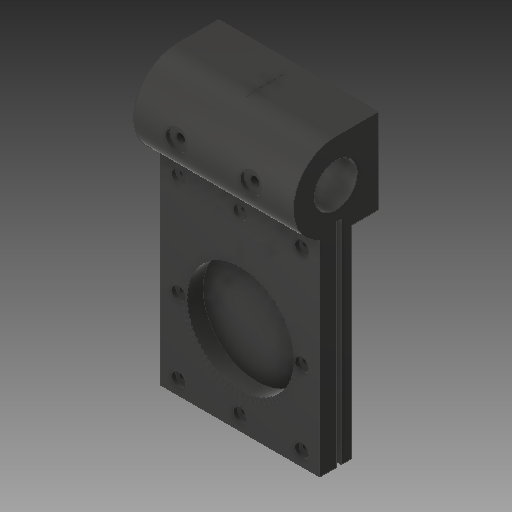
# Autodesk Inventor part: cam_holder_wrist_part
Saved by Autodesk Inventor 2019 (Build 230136000, 136)
## iProperties
Created: 2024-08-06
Part Number: cam_holder_wrist_part
Material: Acetalharz, Schwarz
Document SubType Name: Modeling
Designer: nic
Density: 1.425 g/cm^3
Appearance: Glatt - Schwarz
Author: nic
Autodesk Inventor part; units mm, degrees
(part 1 of 2)
ref_plane "YZ Plane" through (0, 0, 0) normal (1, 0, 0) x (0, 1, 0)
ref_plane "XZ Plane" through (0, 0, 0) normal (0, 1, 0) x (-1, 0, 0)
sketch "Skizze25" plane through (0, 0, 0) normal (1, 0, 0) x (0, 1, 0)
  line L0 (0, 7.5) -> (95, 7.5)
  line L1 (95, -7.5) -> (0, -7.5)
  line L2 (35.3333, -2.65) -> (95, -7.125) construction
  line L3 (100, 0) -> (115, 0) construction
  circle A0 centre (115, 0) radius 10.1
  line L4 (95, -20) -> (135, -20)
  line L5 (135, -20) -> (135, 0)
  line L6 (129.1421, 14.1421) -> (95, -20) construction
  line L7 (100.8579, 14.1421) -> (135, -20) construction
  line L8 (95, -7.125) -> (95, -20)
  line L9 (0, -2.65) -> (100, -2.65)
  line L10 (100, -2.65) -> (100, 2.65)
  line L11 (100, 2.65) -> (0, 2.65)
  line L12 (-100, 2.65) -> (-100, -2.65)
  line L13 (95, 2.5175) -> (100, 2.65) construction
  line L14 (100, -2.65) -> (95, -2.5175) construction
  line L15 (0, 7.5) -> (0, 2.65)
  line L16 (0, -2.65) -> (0, -7.5)
  arc A1 (95.1596, -2.5217) -> (95.1763, -2.65) centre (115, 0) ccw
  line L17 (95, 7.5) -> (96.4595, 7.5)
  arc A2 (135, 0) -> (96.4595, 7.5) centre (115, 0) ccw
  arc A3 (95.1763, 2.65) -> (95.1596, 2.5217) centre (115, 0) ccw
  point P0 (0, 0)
  constraints: 36 end point, 10 point on line, 8 point on circle, 4 centre point, 4 parallel, 3 horizontal, 2 coincident, 1 perpendicular, 1 tangent
extrude "Extrusion21" add sketch "Skizze25" along normal mid plane 75
sketch "Skizze26" plane through (-37.5, 0, 7.5) normal (0, 0, 1) x (1, 0, 0)
  line L0 (37.5, 96.4548) -> (37.5, 41.4548) construction
  circle A0 centre (37.5, 41.4548) radius 25.15
  point P0 (37.5, 0)
  dimension "d109" = 55
  dimension "d110" = 50.3
  constraints: 2 end point, 1 centre point, 1 coincident, 1 vertical
  measures "d109" distance of L0.start L0.end
  measures "d110" diameter of A0
extrude "Extrusion22" cut sketch "Skizze26" against normal up to surface (4.85 mm away)
ref_plane "Arbeitsebene4" through (37.5, 135, 20) normal (0, 0, -1) x (-1, 0, 0)
sketch "Skizze27" plane through (37.5, 135, 20) normal (0, 0, -1) x (-1, 0, 0)
  line L0 (75, -38.5405) -> (0, -38.5405) construction
  line L1 (0, 0) -> (0, -38.5405) construction
  line L2 (75, 0) -> (0, 0) construction
  line L3 (75, -38.5405) -> (75, 0) construction
  line L4 (75, -9.9) -> (75, -30.1) projected
  line L5 (75, -19.2702) -> (0, -19.2702)
  line L6 (75, 0) -> (0, 0) projected
  line L7 (75, 0) -> (55, 0)
  line L8 (0, 0) -> (20, 0)
  point P0 (37.5, -135)
  point P1 (55, -19.2702)
  point P2 (20, -19.2702)
  dimension "d114" = 20
  dimension "d115" = 20
  constraints: 6 end point, 5 point on line, 1 midpoint
  measures "d114" distance of L2.start L7.end
  measures "d115" distance of L1.start L8.end
hole "Bohrung2" at (-17.5, 115.7298, 20) at (17.5, 115.7298, 20) direction (0, 0, -1) diameter 4.2 depth 10 tip angle 118 counterbore diameter 10 counterbore depth 2
sketch "Skizze28" plane through (-37.5, 0, 7.5) normal (0, 0, 1) x (1, 0, 0)
  circle A0 centre (37.5, 41.4548) radius 25.15 construction
  line L0 (8.5, -6.0452) -> (66.5, -6.0452) construction
  line L1 (66.5, -6.0452) -> (66.5, 88.9548) construction
  line L2 (66.5, 88.9548) -> (8.5, 88.9548) construction
  line L3 (8.5, 88.9548) -> (8.5, -6.0452) construction
  line L4 (8.5, -6.0452) -> (66.5, 88.9548) construction
  line L5 (66.5, -6.0452) -> (8.5, 88.9548) construction
  point P0 (37.5, 0)
  point P1 (37.5, 88.9548)
  point P2 (8.5, 41.4548)
  point P3 (66.5, 41.4548)
  point P4 (8.5, 6.4399)
  point P5 (37.5, 6.4399)
  point P6 (66.5, 6.4399)
  dimension "d123" = 58
  dimension "d124" = 95
  constraints: 12 end point, 5 midpoint, 2 coincident, 2 parallel, 2 point on line, 1 horizontal, 1 perpendicular
  measures "d123" distance of L2.end L1.end
  measures "d124" distance of L1.end L0.end
hole "Bohrung3" at (0, 88.9548, 7.5) at (-29, 88.9548, 7.5) at (29, 88.9548, 7.5) at (-29, 41.4548, 7.5) at (29, 41.4548, 7.5) at (-29, 6.4399, 7.5) at (0, 6.4399, 7.5) at (29, 6.4399, 7.5) direction (0, 0, -1) diameter 3.2 end through all counterbore diameter 6.5 counterbore depth 2
sketch "Skizze29" plane through (-37.5, 0, 7.5) normal (0, 0, 1) x (1, 0, 0)
  circle A0 centre (37.5, 41.4548) radius 25.15 projected
  line L0 (37.25, 64.1048) -> (37.75, 64.1048)
  line L1 (37.75, 64.1048) -> (37.75, 69.1048)
  line L2 (37.75, 69.1048) -> (37.25, 69.1048)
  line L3 (37.25, 69.1048) -> (37.25, 64.1048)
  line L4 (37.25, 64.1048) -> (37.75, 69.1048) construction
  line L5 (37.75, 64.1048) -> (37.25, 69.1048) construction
  line L6 (35.2769, 63.9968) -> (35.775, 64.0404)
  line L7 (35.775, 64.0404) -> (35.3392, 69.0214)
  line L8 (35.3392, 69.0214) -> (34.8411, 68.9778)
  line L9 (34.8411, 68.9778) -> (35.2769, 63.9968)
  line L10 (35.2769, 63.9968) -> (35.3392, 69.0214) construction
  line L11 (35.775, 64.0404) -> (34.8411, 68.9778) construction
  line L12 (33.3207, 63.7173) -> (33.8131, 63.8041)
  line L13 (33.8131, 63.8041) -> (32.9448, 68.7282)
  line L14 (32.9448, 68.7282) -> (32.4524, 68.6413)
  line L15 (32.4524, 68.6413) -> (33.3207, 63.7173)
  line L16 (33.3207, 63.7173) -> (32.9448, 68.7282) construction
  line L17 (33.8131, 63.8041) -> (32.4524, 68.6413) construction
  line L18 (31.3963, 63.2683) -> (31.8792, 63.3977)
  line L19 (31.8792, 63.3977) -> (30.5851, 68.2274)
  line L20 (30.5851, 68.2274) -> (30.1022, 68.098)
  line L21 (30.1022, 68.098) -> (31.3963, 63.2683)
  line L22 (31.3963, 63.2683) -> (30.5851, 68.2274) construction
  line L23 (31.8792, 63.3977) -> (30.1022, 68.098) construction
  line L24 (29.5183, 62.6533) -> (29.9882, 62.8244)
  line L25 (29.9882, 62.8244) -> (28.2781, 67.5228)
  line L26 (28.2781, 67.5228) -> (27.8082, 67.3518)
  line L27 (27.8082, 67.3518) -> (29.5183, 62.6533)
  line L28 (29.5183, 62.6533) -> (28.2781, 67.5228) construction
  line L29 (29.9882, 62.8244) -> (27.8082, 67.3518) construction
  line L30 (27.7011, 61.877) -> (28.1543, 62.0883)
  line L31 (28.1543, 62.0883) -> (26.0412, 66.6199)
  line L32 (26.0412, 66.6199) -> (25.588, 66.4086)
  line L33 (25.588, 66.4086) -> (27.7011, 61.877)
  line L34 (27.7011, 61.877) -> (26.0412, 66.6199) construction
  line L35 (28.1543, 62.0883) -> (25.588, 66.4086) construction
  line L36 (25.9585, 60.9453) -> (26.3915, 61.1953)
  line L37 (26.3915, 61.1953) -> (23.8915, 65.5254)
  line L38 (23.8915, 65.5254) -> (23.4585, 65.2754)
  line L39 (23.4585, 65.2754) -> (25.9585, 60.9453)
  line L40 (25.9585, 60.9453) -> (23.8915, 65.5254) construction
  line L41 (26.3915, 61.1953) -> (23.4585, 65.2754) construction
  line L42 (24.3037, 59.8652) -> (24.7133, 60.152)
  line L43 (24.7133, 60.152) -> (21.8454, 64.2478)
  line L44 (21.8454, 64.2478) -> (21.4358, 63.961)
  line L45 (21.4358, 63.961) -> (24.3037, 59.8652)
  line L46 (24.3037, 59.8652) -> (21.8454, 64.2478) construction
  line L47 (24.7133, 60.152) -> (21.4358, 63.961) construction
  line L48 (22.7493, 58.645) -> (23.1324, 58.9664)
  line L49 (23.1324, 58.9664) -> (19.9184, 62.7966)
  line L50 (19.9184, 62.7966) -> (19.5354, 62.4752)
  line L51 (19.5354, 62.4752) -> (22.7493, 58.645)
  line L52 (22.7493, 58.645) -> (19.9184, 62.7966) construction
  line L53 (23.1324, 58.9664) -> (19.5354, 62.4752) construction
  line L54 (21.3073, 57.294) -> (21.6608, 57.6476)
  line L55 (21.6608, 57.6476) -> (18.1253, 61.1831)
  line L56 (18.1253, 61.1831) -> (17.7717, 60.8295)
  line L57 (17.7717, 60.8295) -> (21.3073, 57.294)
  line L58 (21.3073, 57.294) -> (18.1253, 61.1831) construction
  line L59 (21.6608, 57.6476) -> (17.7717, 60.8295) construction
  line L60 (19.9884, 55.8224) -> (20.3098, 56.2055)
  line L61 (20.3098, 56.2055) -> (16.4796, 59.4194)
  line L62 (16.4796, 59.4194) -> (16.1582, 59.0364)
  line L63 (16.1582, 59.0364) -> (19.9884, 55.8224)
  line L64 (19.9884, 55.8224) -> (16.4796, 59.4194) construction
  line L65 (20.3098, 56.2055) -> (16.1582, 59.0364) construction
  line L66 (18.8028, 54.2415) -> (19.0896, 54.6511)
  line L67 (19.0896, 54.6511) -> (14.9938, 57.519)
  line L68 (14.9938, 57.519) -> (14.7071, 57.1094)
  line L69 (14.7071, 57.1094) -> (18.8028, 54.2415)
  line L70 (18.8028, 54.2415) -> (14.9938, 57.519) construction
  line L71 (19.0896, 54.6511) -> (14.7071, 57.1094) construction
  line L72 (17.7595, 52.5633) -> (18.0095, 52.9963)
  line L73 (18.0095, 52.9963) -> (13.6794, 55.4963)
  line L74 (13.6794, 55.4963) -> (13.4294, 55.0633)
  line L75 (13.4294, 55.0633) -> (17.7595, 52.5633)
  line L76 (17.7595, 52.5633) -> (13.6794, 55.4963) construction
  line L77 (18.0095, 52.9963) -> (13.4294, 55.0633) construction
  line L78 (16.8665, 50.8005) -> (17.0778, 51.2537)
  line L79 (17.0778, 51.2537) -> (12.5462, 53.3668)
  line L80 (12.5462, 53.3668) -> (12.3349, 52.9136)
  line L81 (12.3349, 52.9136) -> (16.8665, 50.8005)
  line L82 (16.8665, 50.8005) -> (12.5462, 53.3668) construction
  line L83 (17.0778, 51.2537) -> (12.3349, 52.9136) construction
  line L84 (16.1305, 48.9666) -> (16.3015, 49.4365)
  line L85 (16.3015, 49.4365) -> (11.603, 51.1466)
  line L86 (11.603, 51.1466) -> (11.432, 50.6767)
  line L87 (11.432, 50.6767) -> (16.1305, 48.9666)
  line L88 (16.1305, 48.9666) -> (11.603, 51.1466) construction
  line L89 (16.3015, 49.4365) -> (11.432, 50.6767) construction
  line L90 (15.5571, 47.0756) -> (15.6865, 47.5585)
  line L91 (15.6865, 47.5585) -> (10.8569, 48.8526)
  line L92 (10.8569, 48.8526) -> (10.7274, 48.3697)
  line L93 (10.7274, 48.3697) -> (15.5571, 47.0756)
  line L94 (15.5571, 47.0756) -> (10.8569, 48.8526) construction
  line L95 (15.6865, 47.5585) -> (10.7274, 48.3697) construction
  line L96 (15.1507, 45.1417) -> (15.2375, 45.6341)
  line L97 (15.2375, 45.6341) -> (10.3135, 46.5024)
  line L98 (10.3135, 46.5024) -> (10.2267, 46.01)
  line L99 (10.2267, 46.01) -> (15.1507, 45.1417)
  line L100 (15.1507, 45.1417) -> (10.3135, 46.5024) construction
  line L101 (15.2375, 45.6341) -> (10.2267, 46.01) construction
  line L102 (14.9144, 43.1798) -> (14.958, 43.6779)
  line L103 (14.958, 43.6779) -> (9.977, 44.1137)
  line L104 (9.977, 44.1137) -> (9.9334, 43.6156)
  line L105 (9.9334, 43.6156) -> (14.9144, 43.1798)
  line L106 (14.9144, 43.1798) -> (9.977, 44.1137) construction
  line L107 (14.958, 43.6779) -> (9.9334, 43.6156) construction
  line L108 (14.85, 41.2048) -> (14.85, 41.7048)
  line L109 (14.85, 41.7048) -> (9.85, 41.7048)
  line L110 (9.85, 41.7048) -> (9.85, 41.2048)
  line L111 (9.85, 41.2048) -> (14.85, 41.2048)
  line L112 (14.85, 41.2048) -> (9.85, 41.7048) construction
  line L113 (14.85, 41.7048) -> (9.85, 41.2048) construction
  line L114 (14.958, 39.2317) -> (14.9144, 39.7298)
  line L115 (14.9144, 39.7298) -> (9.9334, 39.294)
  line L116 (9.9334, 39.294) -> (9.977, 38.7959)
  line L117 (9.977, 38.7959) -> (14.958, 39.2317)
  line L118 (14.958, 39.2317) -> (9.9334, 39.294) construction
  line L119 (14.9144, 39.7298) -> (9.977, 38.7959) construction
  line L120 (15.2375, 37.2755) -> (15.1507, 37.7679)
  line L121 (15.1507, 37.7679) -> (10.2267, 36.8996)
  line L122 (10.2267, 36.8996) -> (10.3135, 36.4072)
  line L123 (10.3135, 36.4072) -> (15.2375, 37.2755)
  line L124 (15.2375, 37.2755) -> (10.2267, 36.8996) construction
  line L125 (15.1507, 37.7679) -> (10.3135, 36.4072) construction
  line L126 (15.6865, 35.3511) -> (15.5571, 35.834)
  line L127 (15.5571, 35.834) -> (10.7274, 34.5399)
  line L128 (10.7274, 34.5399) -> (10.8569, 34.057)
  line L129 (10.8569, 34.057) -> (15.6865, 35.3511)
  line L130 (15.6865, 35.3511) -> (10.7274, 34.5399) construction
  line L131 (15.5571, 35.834) -> (10.8569, 34.057) construction
  line L132 (16.3015, 33.4731) -> (16.1305, 33.943)
  line L133 (16.1305, 33.943) -> (11.432, 32.2329)
  line L134 (11.432, 32.2329) -> (11.603, 31.763)
  line L135 (11.603, 31.763) -> (16.3015, 33.4731)
  line L136 (16.3015, 33.4731) -> (11.432, 32.2329) construction
  line L137 (16.1305, 33.943) -> (11.603, 31.763) construction
  line L138 (17.0778, 31.6559) -> (16.8665, 32.1091)
  line L139 (16.8665, 32.1091) -> (12.3349, 29.996)
  line L140 (12.3349, 29.996) -> (12.5462, 29.5428)
  line L141 (12.5462, 29.5428) -> (17.0778, 31.6559)
  line L142 (17.0778, 31.6559) -> (12.3349, 29.996) construction
  line L143 (16.8665, 32.1091) -> (12.5462, 29.5428) construction
  line L144 (18.0095, 29.9133) -> (17.7595, 30.3463)
  line L145 (17.7595, 30.3463) -> (13.4294, 27.8463)
  line L146 (13.4294, 27.8463) -> (13.6794, 27.4133)
  line L147 (13.6794, 27.4133) -> (18.0095, 29.9133)
  line L148 (18.0095, 29.9133) -> (13.4294, 27.8463) construction
  line L149 (17.7595, 30.3463) -> (13.6794, 27.4133) construction
  line L150 (19.0896, 28.2585) -> (18.8028, 28.6681)
  line L151 (18.8028, 28.6681) -> (14.7071, 25.8002)
  line L152 (14.7071, 25.8002) -> (14.9938, 25.3906)
  line L153 (14.9938, 25.3906) -> (19.0896, 28.2585)
  line L154 (19.0896, 28.2585) -> (14.7071, 25.8002) construction
  line L155 (18.8028, 28.6681) -> (14.9938, 25.3906) construction
  line L156 (20.3098, 26.7042) -> (19.9884, 27.0872)
  line L157 (19.9884, 27.0872) -> (16.1582, 23.8732)
  line L158 (16.1582, 23.8732) -> (16.4796, 23.4902)
  line L159 (16.4796, 23.4902) -> (20.3098, 26.7042)
  line L160 (20.3098, 26.7042) -> (16.1582, 23.8732) construction
  line L161 (19.9884, 27.0872) -> (16.4796, 23.4902) construction
  line L162 (21.6608, 25.2621) -> (21.3073, 25.6156)
  line L163 (21.3073, 25.6156) -> (17.7717, 22.0801)
  line L164 (17.7717, 22.0801) -> (18.1253, 21.7265)
  line L165 (18.1253, 21.7265) -> (21.6608, 25.2621)
  line L166 (21.6608, 25.2621) -> (17.7717, 22.0801) construction
  line L167 (21.3073, 25.6156) -> (18.1253, 21.7265) construction
  line L168 (23.1324, 23.9432) -> (22.7493, 24.2646)
  line L169 (22.7493, 24.2646) -> (19.5354, 20.4344)
  line L170 (19.5354, 20.4344) -> (19.9184, 20.113)
  line L171 (19.9184, 20.113) -> (23.1324, 23.9432)
  line L172 (23.1324, 23.9432) -> (19.5354, 20.4344) construction
  line L173 (22.7493, 24.2646) -> (19.9184, 20.113) construction
  line L174 (24.7133, 22.7576) -> (24.3037, 23.0444)
  line L175 (24.3037, 23.0444) -> (21.4358, 18.9486)
  line L176 (21.4358, 18.9486) -> (21.8454, 18.6619)
  line L177 (21.8454, 18.6619) -> (24.7133, 22.7576)
  line L178 (24.7133, 22.7576) -> (21.4358, 18.9486) construction
  line L179 (24.3037, 23.0444) -> (21.8454, 18.6619) construction
  line L180 (26.3915, 21.7143) -> (25.9585, 21.9643)
  line L181 (25.9585, 21.9643) -> (23.4585, 17.6342)
  line L182 (23.4585, 17.6342) -> (23.8915, 17.3842)
  line L183 (23.8915, 17.3842) -> (26.3915, 21.7143)
  line L184 (26.3915, 21.7143) -> (23.4585, 17.6342) construction
  line L185 (25.9585, 21.9643) -> (23.8915, 17.3842) construction
  line L186 (28.1543, 20.8213) -> (27.7011, 21.0326)
  line L187 (27.7011, 21.0326) -> (25.588, 16.5011)
  line L188 (25.588, 16.5011) -> (26.0412, 16.2897)
  line L189 (26.0412, 16.2897) -> (28.1543, 20.8213)
  line L190 (28.1543, 20.8213) -> (25.588, 16.5011) construction
  line L191 (27.7011, 21.0326) -> (26.0412, 16.2897) construction
  line L192 (29.9882, 20.0853) -> (29.5183, 20.2563)
  line L193 (29.5183, 20.2563) -> (27.8082, 15.5578)
  line L194 (27.8082, 15.5578) -> (28.2781, 15.3868)
  line L195 (28.2781, 15.3868) -> (29.9882, 20.0853)
  line L196 (29.9882, 20.0853) -> (27.8082, 15.5578) construction
  line L197 (29.5183, 20.2563) -> (28.2781, 15.3868) construction
  line L198 (31.8792, 19.5119) -> (31.3963, 19.6413)
  line L199 (31.3963, 19.6413) -> (30.1022, 14.8117)
  line L200 (30.1022, 14.8117) -> (30.5851, 14.6823)
  line L201 (30.5851, 14.6823) -> (31.8792, 19.5119)
  line L202 (31.8792, 19.5119) -> (30.1022, 14.8117) construction
  line L203 (31.3963, 19.6413) -> (30.5851, 14.6823) construction
  line L204 (33.8131, 19.1055) -> (33.3207, 19.1923)
  line L205 (33.3207, 19.1923) -> (32.4524, 14.2683)
  line L206 (32.4524, 14.2683) -> (32.9448, 14.1815)
  line L207 (32.9448, 14.1815) -> (33.8131, 19.1055)
  line L208 (33.8131, 19.1055) -> (32.4524, 14.2683) construction
  line L209 (33.3207, 19.1923) -> (32.9448, 14.1815) construction
  line L210 (35.775, 18.8692) -> (35.2769, 18.9128)
  line L211 (35.2769, 18.9128) -> (34.8411, 13.9318)
  line L212 (34.8411, 13.9318) -> (35.3392, 13.8882)
  line L213 (35.3392, 13.8882) -> (35.775, 18.8692)
  line L214 (35.775, 18.8692) -> (34.8411, 13.9318) construction
  line L215 (35.2769, 18.9128) -> (35.3392, 13.8882) construction
  line L216 (37.75, 18.8048) -> (37.25, 18.8048)
  line L217 (37.25, 18.8048) -> (37.25, 13.8048)
  line L218 (37.25, 13.8048) -> (37.75, 13.8048)
  line L219 (37.75, 13.8048) -> (37.75, 18.8048)
  line L220 (37.75, 18.8048) -> (37.25, 13.8048) construction
  line L221 (37.25, 18.8048) -> (37.75, 13.8048) construction
  line L222 (39.7231, 18.9128) -> (39.225, 18.8692)
  line L223 (39.225, 18.8692) -> (39.6608, 13.8882)
  line L224 (39.6608, 13.8882) -> (40.1589, 13.9318)
  line L225 (40.1589, 13.9318) -> (39.7231, 18.9128)
  line L226 (39.7231, 18.9128) -> (39.6608, 13.8882) construction
  line L227 (39.225, 18.8692) -> (40.1589, 13.9318) construction
  line L228 (41.6793, 19.1923) -> (41.1869, 19.1055)
  line L229 (41.1869, 19.1055) -> (42.0552, 14.1815)
  line L230 (42.0552, 14.1815) -> (42.5476, 14.2683)
  line L231 (42.5476, 14.2683) -> (41.6793, 19.1923)
  line L232 (41.6793, 19.1923) -> (42.0552, 14.1815) construction
  line L233 (41.1869, 19.1055) -> (42.5476, 14.2683) construction
  line L234 (43.6037, 19.6413) -> (43.1208, 19.5119)
  line L235 (43.1208, 19.5119) -> (44.4149, 14.6823)
  line L236 (44.4149, 14.6823) -> (44.8978, 14.8117)
  line L237 (44.8978, 14.8117) -> (43.6037, 19.6413)
  line L238 (43.6037, 19.6413) -> (44.4149, 14.6823) construction
  line L239 (43.1208, 19.5119) -> (44.8978, 14.8117) construction
  line L240 (45.4817, 20.2563) -> (45.0118, 20.0853)
  line L241 (45.0118, 20.0853) -> (46.7219, 15.3868)
  line L242 (46.7219, 15.3868) -> (47.1918, 15.5578)
  line L243 (47.1918, 15.5578) -> (45.4817, 20.2563)
  line L244 (45.4817, 20.2563) -> (46.7219, 15.3868) construction
  line L245 (45.0118, 20.0853) -> (47.1918, 15.5578) construction
  line L246 (47.2989, 21.0326) -> (46.8457, 20.8213)
  line L247 (46.8457, 20.8213) -> (48.9588, 16.2897)
  line L248 (48.9588, 16.2897) -> (49.412, 16.5011)
  line L249 (49.412, 16.5011) -> (47.2989, 21.0326)
  line L250 (47.2989, 21.0326) -> (48.9588, 16.2897) construction
  line L251 (46.8457, 20.8213) -> (49.412, 16.5011) construction
  line L252 (49.0415, 21.9643) -> (48.6085, 21.7143)
  line L253 (48.6085, 21.7143) -> (51.1085, 17.3842)
  line L254 (51.1085, 17.3842) -> (51.5415, 17.6342)
  line L255 (51.5415, 17.6342) -> (49.0415, 21.9643)
  line L256 (49.0415, 21.9643) -> (51.1085, 17.3842) construction
  line L257 (48.6085, 21.7143) -> (51.5415, 17.6342) construction
  line L258 (50.6963, 23.0444) -> (50.2867, 22.7576)
  line L259 (50.2867, 22.7576) -> (53.1546, 18.6619)
  line L260 (53.1546, 18.6619) -> (53.5642, 18.9486)
  line L261 (53.5642, 18.9486) -> (50.6963, 23.0444)
  line L262 (50.6963, 23.0444) -> (53.1546, 18.6619) construction
  line L263 (50.2867, 22.7576) -> (53.5642, 18.9486) construction
  line L264 (52.2507, 24.2646) -> (51.8676, 23.9432)
  line L265 (51.8676, 23.9432) -> (55.0816, 20.113)
  line L266 (55.0816, 20.113) -> (55.4646, 20.4344)
  line L267 (55.4646, 20.4344) -> (52.2507, 24.2646)
  line L268 (52.2507, 24.2646) -> (55.0816, 20.113) construction
  line L269 (51.8676, 23.9432) -> (55.4646, 20.4344) construction
  line L270 (53.6927, 25.6156) -> (53.3392, 25.2621)
  line L271 (53.3392, 25.2621) -> (56.8747, 21.7265)
  line L272 (56.8747, 21.7265) -> (57.2283, 22.0801)
  line L273 (57.2283, 22.0801) -> (53.6927, 25.6156)
  line L274 (53.6927, 25.6156) -> (56.8747, 21.7265) construction
  line L275 (53.3392, 25.2621) -> (57.2283, 22.0801) construction
  line L276 (55.0116, 27.0872) -> (54.6902, 26.7042)
  line L277 (54.6902, 26.7042) -> (58.5204, 23.4902)
  line L278 (58.5204, 23.4902) -> (58.8418, 23.8732)
  line L279 (58.8418, 23.8732) -> (55.0116, 27.0872)
  line L280 (55.0116, 27.0872) -> (58.5204, 23.4902) construction
  line L281 (54.6902, 26.7042) -> (58.8418, 23.8732) construction
  line L282 (56.1972, 28.6681) -> (55.9104, 28.2585)
  line L283 (55.9104, 28.2585) -> (60.0062, 25.3906)
  line L284 (60.0062, 25.3906) -> (60.2929, 25.8002)
  line L285 (60.2929, 25.8002) -> (56.1972, 28.6681)
  line L286 (56.1972, 28.6681) -> (60.0062, 25.3906) construction
  line L287 (55.9104, 28.2585) -> (60.2929, 25.8002) construction
  line L288 (57.2405, 30.3463) -> (56.9905, 29.9133)
  line L289 (56.9905, 29.9133) -> (61.3206, 27.4133)
  line L290 (61.3206, 27.4133) -> (61.5706, 27.8463)
  line L291 (61.5706, 27.8463) -> (57.2405, 30.3463)
  line L292 (57.2405, 30.3463) -> (61.3206, 27.4133) construction
  line L293 (56.9905, 29.9133) -> (61.5706, 27.8463) construction
  line L294 (58.1335, 32.1091) -> (57.9222, 31.6559)
  line L295 (57.9222, 31.6559) -> (62.4538, 29.5428)
  line L296 (62.4538, 29.5428) -> (62.6651, 29.996)
  line L297 (62.6651, 29.996) -> (58.1335, 32.1091)
  line L298 (58.1335, 32.1091) -> (62.4538, 29.5428) construction
  line L299 (57.9222, 31.6559) -> (62.6651, 29.996) construction
  line L300 (58.8695, 33.943) -> (58.6985, 33.4731)
  line L301 (58.6985, 33.4731) -> (63.397, 31.763)
  line L302 (63.397, 31.763) -> (63.568, 32.2329)
  line L303 (63.568, 32.2329) -> (58.8695, 33.943)
  line L304 (58.8695, 33.943) -> (63.397, 31.763) construction
  line L305 (58.6985, 33.4731) -> (63.568, 32.2329) construction
  line L306 (59.4429, 35.834) -> (59.3135, 35.3511)
  line L307 (59.3135, 35.3511) -> (64.1431, 34.057)
  line L308 (64.1431, 34.057) -> (64.2726, 34.5399)
  line L309 (64.2726, 34.5399) -> (59.4429, 35.834)
  line L310 (59.4429, 35.834) -> (64.1431, 34.057) construction
  line L311 (59.3135, 35.3511) -> (64.2726, 34.5399) construction
  line L312 (59.8493, 37.7679) -> (59.7625, 37.2755)
  line L313 (59.7625, 37.2755) -> (64.6865, 36.4072)
  line L314 (64.6865, 36.4072) -> (64.7733, 36.8996)
  line L315 (64.7733, 36.8996) -> (59.8493, 37.7679)
  line L316 (59.8493, 37.7679) -> (64.6865, 36.4072) construction
  line L317 (59.7625, 37.2755) -> (64.7733, 36.8996) construction
  line L318 (60.0856, 39.7298) -> (60.042, 39.2317)
  line L319 (60.042, 39.2317) -> (65.023, 38.7959)
  line L320 (65.023, 38.7959) -> (65.0666, 39.294)
  line L321 (65.0666, 39.294) -> (60.0856, 39.7298)
  line L322 (60.0856, 39.7298) -> (65.023, 38.7959) construction
  line L323 (60.042, 39.2317) -> (65.0666, 39.294) construction
  line L324 (60.15, 41.7048) -> (60.15, 41.2048)
  line L325 (60.15, 41.2048) -> (65.15, 41.2048)
  line L326 (65.15, 41.2048) -> (65.15, 41.7048)
  line L327 (65.15, 41.7048) -> (60.15, 41.7048)
  line L328 (60.15, 41.7048) -> (65.15, 41.2048) construction
  line L329 (60.15, 41.2048) -> (65.15, 41.7048) construction
  line L330 (60.042, 43.6779) -> (60.0856, 43.1798)
  line L331 (60.0856, 43.1798) -> (65.0666, 43.6156)
  line L332 (65.0666, 43.6156) -> (65.023, 44.1137)
  line L333 (65.023, 44.1137) -> (60.042, 43.6779)
  line L334 (60.042, 43.6779) -> (65.0666, 43.6156) construction
  line L335 (60.0856, 43.1798) -> (65.023, 44.1137) construction
  line L336 (59.7625, 45.6341) -> (59.8493, 45.1417)
  line L337 (59.8493, 45.1417) -> (64.7733, 46.01)
  line L338 (64.7733, 46.01) -> (64.6865, 46.5024)
  line L339 (64.6865, 46.5024) -> (59.7625, 45.6341)
  line L340 (59.7625, 45.6341) -> (64.7733, 46.01) construction
  line L341 (59.8493, 45.1417) -> (64.6865, 46.5024) construction
  line L342 (59.3135, 47.5585) -> (59.4429, 47.0756)
  line L343 (59.4429, 47.0756) -> (64.2726, 48.3697)
  line L344 (64.2726, 48.3697) -> (64.1431, 48.8526)
  line L345 (64.1431, 48.8526) -> (59.3135, 47.5585)
  line L346 (59.3135, 47.5585) -> (64.2726, 48.3697) construction
  line L347 (59.4429, 47.0756) -> (64.1431, 48.8526) construction
  line L348 (58.6985, 49.4365) -> (58.8695, 48.9666)
  line L349 (58.8695, 48.9666) -> (63.568, 50.6767)
  line L350 (63.568, 50.6767) -> (63.397, 51.1466)
  line L351 (63.397, 51.1466) -> (58.6985, 49.4365)
  line L352 (58.6985, 49.4365) -> (63.568, 50.6767) construction
  line L353 (58.8695, 48.9666) -> (63.397, 51.1466) construction
  line L354 (57.9222, 51.2537) -> (58.1335, 50.8005)
  line L355 (58.1335, 50.8005) -> (62.6651, 52.9136)
  line L356 (62.6651, 52.9136) -> (62.4538, 53.3668)
  line L357 (62.4538, 53.3668) -> (57.9222, 51.2537)
  line L358 (57.9222, 51.2537) -> (62.6651, 52.9136) construction
  line L359 (58.1335, 50.8005) -> (62.4538, 53.3668) construction
  line L360 (56.9905, 52.9963) -> (57.2405, 52.5633)
  line L361 (57.2405, 52.5633) -> (61.5706, 55.0633)
  line L362 (61.5706, 55.0633) -> (61.3206, 55.4963)
  line L363 (61.3206, 55.4963) -> (56.9905, 52.9963)
  line L364 (56.9905, 52.9963) -> (61.5706, 55.0633) construction
  line L365 (57.2405, 52.5633) -> (61.3206, 55.4963) construction
  line L366 (55.9104, 54.6511) -> (56.1972, 54.2415)
  line L367 (56.1972, 54.2415) -> (60.2929, 57.1094)
  line L368 (60.2929, 57.1094) -> (60.0062, 57.519)
  line L369 (60.0062, 57.519) -> (55.9104, 54.6511)
  line L370 (55.9104, 54.6511) -> (60.2929, 57.1094) construction
  line L371 (56.1972, 54.2415) -> (60.0062, 57.519) construction
  line L372 (54.6902, 56.2055) -> (55.0116, 55.8224)
  line L373 (55.0116, 55.8224) -> (58.8418, 59.0364)
  line L374 (58.8418, 59.0364) -> (58.5204, 59.4194)
  line L375 (58.5204, 59.4194) -> (54.6902, 56.2055)
  line L376 (54.6902, 56.2055) -> (58.8418, 59.0364) construction
  line L377 (55.0116, 55.8224) -> (58.5204, 59.4194) construction
  line L378 (53.3392, 57.6476) -> (53.6927, 57.294)
  line L379 (53.6927, 57.294) -> (57.2283, 60.8295)
  line L380 (57.2283, 60.8295) -> (56.8747, 61.1831)
  line L381 (56.8747, 61.1831) -> (53.3392, 57.6476)
  line L382 (53.3392, 57.6476) -> (57.2283, 60.8295) construction
  line L383 (53.6927, 57.294) -> (56.8747, 61.1831) construction
  line L384 (51.8676, 58.9664) -> (52.2507, 58.645)
  line L385 (52.2507, 58.645) -> (55.4646, 62.4752)
  line L386 (55.4646, 62.4752) -> (55.0816, 62.7966)
  line L387 (55.0816, 62.7966) -> (51.8676, 58.9664)
  line L388 (51.8676, 58.9664) -> (55.4646, 62.4752) construction
  line L389 (52.2507, 58.645) -> (55.0816, 62.7966) construction
  line L390 (50.2867, 60.152) -> (50.6963, 59.8652)
  line L391 (50.6963, 59.8652) -> (53.5642, 63.961)
  line L392 (53.5642, 63.961) -> (53.1546, 64.2478)
  line L393 (53.1546, 64.2478) -> (50.2867, 60.152)
  line L394 (50.2867, 60.152) -> (53.5642, 63.961) construction
  line L395 (50.6963, 59.8652) -> (53.1546, 64.2478) construction
  line L396 (48.6085, 61.1953) -> (49.0415, 60.9453)
  line L397 (49.0415, 60.9453) -> (51.5415, 65.2754)
  line L398 (51.5415, 65.2754) -> (51.1085, 65.5254)
  line L399 (51.1085, 65.5254) -> (48.6085, 61.1953)
  line L400 (48.6085, 61.1953) -> (51.5415, 65.2754) construction
  line L401 (49.0415, 60.9453) -> (51.1085, 65.5254) construction
  line L402 (46.8457, 62.0883) -> (47.2989, 61.877)
  line L403 (47.2989, 61.877) -> (49.412, 66.4086)
  line L404 (49.412, 66.4086) -> (48.9588, 66.6199)
  line L405 (48.9588, 66.6199) -> (46.8457, 62.0883)
  line L406 (46.8457, 62.0883) -> (49.412, 66.4086) construction
  line L407 (47.2989, 61.877) -> (48.9588, 66.6199) construction
  line L408 (45.0118, 62.8244) -> (45.4817, 62.6533)
  line L409 (45.4817, 62.6533) -> (47.1918, 67.3518)
  line L410 (47.1918, 67.3518) -> (46.7219, 67.5228)
  line L411 (46.7219, 67.5228) -> (45.0118, 62.8244)
  line L412 (45.0118, 62.8244) -> (47.1918, 67.3518) construction
  line L413 (45.4817, 62.6533) -> (46.7219, 67.5228) construction
  line L414 (43.1208, 63.3977) -> (43.6037, 63.2683)
  line L415 (43.6037, 63.2683) -> (44.8978, 68.098)
  line L416 (44.8978, 68.098) -> (44.4149, 68.2274)
  line L417 (44.4149, 68.2274) -> (43.1208, 63.3977)
  line L418 (43.1208, 63.3977) -> (44.8978, 68.098) construction
  line L419 (43.6037, 63.2683) -> (44.4149, 68.2274) construction
  line L420 (41.1869, 63.8041) -> (41.6793, 63.7173)
  line L421 (41.6793, 63.7173) -> (42.5476, 68.6413)
  line L422 (42.5476, 68.6413) -> (42.0552, 68.7282)
  line L423 (42.0552, 68.7282) -> (41.1869, 63.8041)
  line L424 (41.1869, 63.8041) -> (42.5476, 68.6413) construction
  line L425 (41.6793, 63.7173) -> (42.0552, 68.7282) construction
  line L426 (39.225, 64.0404) -> (39.7231, 63.9968)
  line L427 (39.7231, 63.9968) -> (40.1589, 68.9778)
  line L428 (40.1589, 68.9778) -> (39.6608, 69.0214)
  line L429 (39.6608, 69.0214) -> (39.225, 64.0404)
  line L430 (39.225, 64.0404) -> (40.1589, 68.9778) construction
  line L431 (39.7231, 63.9968) -> (39.6608, 69.0214) construction
  line L432 (37.75, 7.3607) -> (37.25, 7.3607)
  line L433 (37.25, 7.3607) -> (37.25, 75.5489)
  line L434 (37.25, 75.5489) -> (37.75, 75.5489)
  line L435 (37.75, 75.5489) -> (37.75, 7.3607)
  line L436 (37.75, 7.3607) -> (37.25, 75.5489) construction
  line L437 (37.25, 7.3607) -> (37.75, 75.5489) construction
  point P0 (37.5, 0)
  point P1 (37.5, 66.6048)
  point P2 (35.308, 66.5091)
  point P3 (33.1327, 66.2227)
  point P4 (30.9907, 65.7478)
  point P5 (28.8982, 65.0881)
  point P6 (26.8712, 64.2484)
  point P7 (24.925, 63.2353)
  point P8 (23.0746, 62.0565)
  point P9 (21.3339, 60.7208)
  point P10 (19.7163, 59.2385)
  point P11 (18.234, 57.6209)
  point P12 (16.8983, 55.8803)
  point P13 (15.7195, 54.0298)
  point P14 (14.7064, 52.0837)
  point P15 (13.8667, 50.0566)
  point P16 (13.207, 47.9641)
  point P17 (12.7321, 45.8221)
  point P18 (12.4457, 43.6468)
  point P19 (12.35, 41.4548)
  point P20 (12.4457, 39.2628)
  point P21 (12.7321, 37.0876)
  point P22 (13.207, 34.9455)
  point P23 (13.8667, 32.853)
  point P24 (14.7064, 30.826)
  point P25 (15.7195, 28.8798)
  point P26 (16.8983, 27.0294)
  point P27 (18.234, 25.2887)
  point P28 (19.7163, 23.6711)
  point P29 (21.3339, 22.1888)
  point P30 (23.0746, 20.8531)
  point P31 (24.925, 19.6743)
  point P32 (26.8712, 18.6612)
  point P33 (28.8982, 17.8215)
  point P34 (30.9907, 17.1618)
  point P35 (33.1327, 16.6869)
  point P36 (35.308, 16.4005)
  point P37 (37.5, 16.3048)
  point P38 (39.692, 16.4005)
  point P39 (41.8673, 16.6869)
  point P40 (44.0093, 17.1618)
  point P41 (46.1018, 17.8215)
  point P42 (48.1288, 18.6612)
  point P43 (50.075, 19.6743)
  point P44 (51.9254, 20.8531)
  point P45 (53.6661, 22.1888)
  point P46 (55.2837, 23.6711)
  point P47 (56.766, 25.2887)
  point P48 (58.1017, 27.0294)
  point P49 (59.2805, 28.8798)
  point P50 (60.2936, 30.826)
  point P51 (61.1333, 32.853)
  point P52 (61.793, 34.9455)
  point P53 (62.2679, 37.0876)
  point P54 (62.5543, 39.2628)
  point P55 (62.65, 41.4548)
  point P56 (62.5543, 43.6468)
  point P57 (62.2679, 45.8221)
  point P58 (61.793, 47.9641)
  point P59 (61.1333, 50.0566)
  point P60 (60.2936, 52.0837)
  point P61 (59.2805, 54.0298)
  point P62 (58.1017, 55.8803)
  point P63 (56.766, 57.6209)
  point P64 (55.2837, 59.2385)
  point P65 (53.6661, 60.7208)
  point P66 (51.9254, 62.0565)
  point P67 (50.075, 63.2353)
  point P68 (48.1288, 64.2484)
  point P69 (46.1018, 65.0881)
  point P70 (44.0093, 65.7478)
  point P71 (41.8673, 66.2227)
  point P72 (39.692, 66.5091)
  dimension "d132" = 0.5
  dimension "d133" = 5
  dimension "d136" = 360
  dimension "d138" = 0.5
  constraints: 876 end point, 146 midpoint, 4 parallel, 2 horizontal, 2 perpendicular, 1 vertical alignment, 794 other
  measures "d132" distance of L2.end L1.end
  measures "d133" distance of L1.end L0.end
  measures "d138" distance of L433.end L434.end
extrude "Extrusion23" cut sketch "Skizze29" against normal blind 0.5 contours A0 L325 L324 L327 | A0 L327 L326 L325 | L331 L330 L333 A0 | A0 L333 L332 L331 | L321 L320 L319 A0 | A0 L319 L318 L321 | L337 L336 L339 A0 | A0 L339 L338 L337 | L315 L314 L313 A0 | A0 L313 L312 L315 | L343 L342 L345 A0 | A0 L345 L344 L343 | L309 L308 L307 A0 | A0 L307 L306 L309 | L349 L348 L351 A0 | A0 L351 L350 L349 | L303 L302 L301 A0 | A0 L301 L300 L303 | L355 L354 L357 A0 | A0 L357 L356 L355 | L297 L296 L295 A0 | A0 L295 L294 L297 | L361 L360 L363 A0 | A0 L363 L362 L361 | L291 L290 L289 A0 | A0 L289 L288 L291 | L367 L366 L369 A0 | A0 L369 L368 L367 | L285 L284 L283 A0 | A0 L283 L282 L285 | L373 L372 L375 A0 | A0 L375 L374 L373 | L279 L278 L277 A0 | A0 L277 L276 L279 | L379 L378 L381 A0 | A0 L381 L380 L379 | L273 L272 L271 A0 | A0 L271 L270 L273 | L385 L384 L387 A0 | A0 L387 L386 L385 | L267 L266 L265 A0 | A0 L265 L264 L267 | L391 L390 L393 A0 | A0 L393 L392 L391 | L261 L260 L259 A0 | A0 L259 L258 L261 | L397 L396 L399 A0 | A0 L399 L398 L397 | L255 L254 L253 A0 | A0 L253 L252 L255 | L403 L402 L405 A0 | A0 L405 L404 L403 | L249 L248 L247 A0 | A0 L247 L246 L249 | L409 L408 L411 A0 | A0 L411 L410 L409 | L243 L242 L241 A0 | A0 L241 L240 L243 | L415 L414 L417 A0 | A0 L417 L416 L415 | L237 L236 L235 A0 | A0 L235 L234 L237 | L421 L420 L423 A0 | A0 L423 L422 L421 | L231 L230 L229 A0 | A0 L229 L228 L231 | L427 L426 L429 A0 | A0 L429 L428 L427 | L225 L224 L223 A0 | A0 L223 L222 L225 | L1 L0 L3 A0 | A0 L3 L2 L1 | L219 L218 L217 A0 | A0 L217 L216 L219 | L435 L216 L433 L0 | L2 L433 L434 L435 | L435 L432 L433 L218 | L7 L6 L9 A0 | A0 L9 L8 L7 | L213 L212 L211 A0 | A0 L211 L210 L213 | L13 L12 L15 A0 | A0 L15 L14 L13 | L207 L206 L205 A0 | A0 L205 L204 L207 | L19 L18 L21 A0 | A0 L21 L20 L19 | L201 L200 L199 A0 | A0 L199 L198 L201 | L25 L24 L27 A0 | A0 L27 L26 L25 | L195 L194 L193 A0 | A0 L193 L192 L195 | L31 L30 L33 A0 | A0 L33 L32 L31 | L189 L188 L187 A0 | A0 L187 L186 L189 | L37 L36 L39 A0 | A0 L39 L38 L37 | L183 L182 L181 A0 | A0 L181 L180 L183 | L43 L42 L45 A0 | A0 L45 L44 L43 | L177 L176 L175 A0 | A0 L175 L174 L177 | L49 L48 L51 A0 | A0 L51 L50 L49 | L171 L170 L169 A0 | A0 L169 L168 L171 | L55 L54 L57 A0 | A0 L57 L56 L55 | L165 L164 L163 A0 | A0 L163 L162 L165 | L61 L60 L63 A0 | A0 L63 L62 L61 | L159 L158 L157 A0 | A0 L157 L156 L159 | L67 L66 L69 A0 | A0 L69 L68 L67 | L153 L152 L151 A0 | A0 L151 L150 L153 | L73 L72 L75 A0 | A0 L75 L74 L73 | L147 L146 L145 A0 | A0 L145 L144 L147 | L79 L78 L81 A0 | A0 L81 L80 L79 | L141 L140 L139 A0 | A0 L139 L138 L141 | L85 L84 L87 A0 | A0 L87 L86 L85 | L135 L134 L133 A0 | A0 L133 L132 L135 | L91 L90 L93 A0 | A0 L93 L92 L91 | L129 L128 L127 A0 | A0 L127 L126 L129 | L97 L96 L99 A0 | A0 L99 L98 L97 | L123 L122 L121 A0 | A0 L121 L120 L123 | L103 L102 L105 A0 | A0 L105 L104 L103 | L117 L116 L115 A0 | A0 L115 L114 L117 | L109 L108 L111 A0 | A0 L111 L110 L109
sketch "Skizze30" plane through (-37.5, 0, 7.5) normal (0, 0, 1) x (1, 0, 0)
  line L0 (50.276, 82.0666) -> (69.0257, 82.0666) construction
  line L1 (69.0257, 82.0666) -> (69.0257, 69.013) construction
  line L2 (69.0257, 69.013) -> (50.276, 69.013) construction
  line L3 (50.276, 69.013) -> (50.276, 82.0666) construction
  spline S0 degree 2 poles (52.6528, 79.6189) (52.6528, 79.3664) (52.4911, 78.9353) (52.3436, 78.7765) knots 0 0 0 1 2 2 2
  spline S1 degree 2 poles (52.3436, 78.7765) (52.1961, 78.6176) (51.7565, 78.4333) (51.4842, 78.4333) knots 0 0 0 1 2 2 2
  spline S2 degree 2 poles (51.4842, 78.4333) (51.2346, 78.4333) (50.7468, 78.5439) (50.5681, 78.6318) knots 0 0 0 1 2 2 2
  line L4 (50.5681, 78.6318) -> (50.5681, 79.1282)
  line L5 (50.5681, 79.1282) -> (50.6021, 79.1282)
  spline S3 degree 2 poles (50.6021, 79.1282) (50.656, 79.0885) (50.8574, 78.9864) (50.9794, 78.941) knots 0 0 0 1 2 2 2
  spline S4 degree 2 poles (50.9794, 78.941) (51.1184, 78.8928) (51.3481, 78.8389) (51.4927, 78.8389) knots 0 0 0 1 2 2 2
  spline S5 degree 2 poles (51.4927, 78.8389) (51.6346, 78.8389) (51.9012, 78.941) (51.9976, 79.0516) knots 0 0 0 1 2 2 2
  spline S6 degree 2 poles (51.9976, 79.0516) (52.0855, 79.1565) (52.1763, 79.4345) (52.1763, 79.6217) knots 0 0 0 1 2 2 2
  spline S7 degree 2 poles (52.1763, 79.6217) (52.1763, 79.8089) (52.0742, 80.0471) (51.9778, 80.1266) knots 0 0 0 1 2 2 2
  spline S8 degree 2 poles (51.9778, 80.1266) (51.8785, 80.2145) (51.5835, 80.2882) (51.4048, 80.2882) knots 0 0 0 1 2 2 2
  spline S9 degree 2 poles (51.4048, 80.2882) (51.212, 80.2882) (50.8291, 80.2287) (50.7128, 80.2031) knots 0 0 0 1 2 2 2
  line L6 (50.7128, 80.2031) -> (50.7128, 82.007)
  line L7 (50.7128, 82.007) -> (52.6329, 82.007)
  line L8 (52.6329, 82.007) -> (52.6329, 81.5958)
  line L9 (52.6329, 81.5958) -> (51.1637, 81.5958)
  line L10 (51.1637, 81.5958) -> (51.1637, 80.6626)
  spline S10 degree 2 poles (51.1637, 80.6626) (51.2488, 80.674) (51.4133, 80.6825) (51.4814, 80.6825) knots 0 0 0 1 2 2 2
  spline S11 degree 2 poles (51.4814, 80.6825) (51.7508, 80.6825) (52.1224, 80.5946) (52.2926, 80.4641) knots 0 0 0 1 2 2 2
  spline S12 degree 2 poles (52.2926, 80.4641) (52.4656, 80.3336) (52.6528, 79.9365) (52.6528, 79.6189) knots 0 0 0 1 2 2 2
  spline S13 degree 2 poles (54.9303, 81.1732) (54.9303, 80.7959) (54.4141, 80.2797) (54.0369, 80.2797) knots 0 0 0 1 2 2 2
  spline S14 degree 2 poles (54.0369, 80.2797) (53.6625, 80.2797) (53.1406, 80.7931) (53.1406, 81.1732) knots 0 0 0 1 2 2 2
  spline S15 degree 2 poles (53.1406, 81.1732) (53.1406, 81.5504) (53.6568, 82.0666) (54.0369, 82.0666) knots 0 0 0 1 2 2 2
  spline S16 degree 2 poles (54.0369, 82.0666) (54.4141, 82.0666) (54.9303, 81.5504) (54.9303, 81.1732) knots 0 0 0 1 2 2 2
  spline S17 degree 2 poles (54.5616, 81.1732) (54.5616, 81.4001) (54.261, 81.7092) (54.0369, 81.7092) knots 0 0 0 1 2 2 2
  spline S18 degree 2 poles (54.0369, 81.7092) (53.81, 81.7092) (53.5094, 81.4001) (53.5094, 81.1732) knots 0 0 0 1 2 2 2
  spline S19 degree 2 poles (53.5094, 81.1732) (53.5094, 80.9434) (53.8157, 80.6371) (54.0369, 80.6371) knots 0 0 0 1 2 2 2
  spline S20 degree 2 poles (54.0369, 80.6371) (54.261, 80.6371) (54.5616, 80.9491) (54.5616, 81.1732) knots 0 0 0 1 2 2 2
  point P0 (37.5, 0)
  constraints: 2 other
extrude "Extrusion24" cut sketch "Skizze30" against normal blind 0.5